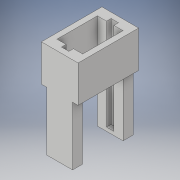
# Autodesk Inventor part: Colorimeter_Mounting-Tool
Saved by Autodesk Inventor 2019 (Build 230136000, 136)
## iProperties
Created: 2019-04-03
Part Number: Colorimeter_Mounting-Tool
Material: Generic
Document SubType Name: Modeling
Designer: Hansen
Density: 1 g/cm^3
Appearance: Default
Author: Hansen
Autodesk Inventor part; units mm, degrees
ref_plane "YZ Plane" through (0, 0, 0) normal (1, 0, 0) x (0, 1, 0)
ref_plane "XZ Plane" through (0, 0, 0) normal (0, 1, 0) x (-1, 0, 0)
ref_plane "XY Plane" through (0, 0, 0) normal (0, 0, 1) x (1, 0, 0)
sketch "Sketch1" plane through (0, 0, 0) normal (0, 1, 0) x (-1, 0, 0)
  line L0 (1, 6.75) -> (3.5, 6.75)
  line L1 (3.5, 6.75) -> (3.5, 5.5)
  line L2 (3.5, 5.5) -> (1, 5.5)
  line L3 (1, 5.5) -> (1, 6.75)
  line L4 (1, 6.75) -> (3.5, 5.5) construction
  line L5 (3.5, 6.75) -> (1, 5.5) construction
  line L6 (1, -5.5) -> (3.5, -5.5)
  line L7 (3.5, -5.5) -> (3.5, -6.75)
  line L8 (3.5, -6.75) -> (1, -6.75)
  line L9 (1, -6.75) -> (1, -5.5)
  line L10 (1, -5.5) -> (3.5, -6.75) construction
  line L11 (3.5, -5.5) -> (1, -6.75) construction
  line L12 (-1, 6.75) -> (-3.5, 6.75)
  line L13 (-3.5, 6.75) -> (-3.5, 5.5)
  line L14 (-3.5, 5.5) -> (-1, 5.5)
  line L15 (-1, 5.5) -> (-1, 6.75)
  line L16 (-1, 6.75) -> (-3.5, 5.5) construction
  line L17 (-3.5, 6.75) -> (-1, 5.5) construction
  line L18 (-1, -5.5) -> (-3.5, -5.5)
  line L19 (-3.5, -5.5) -> (-3.5, -6.75)
  line L20 (-3.5, -6.75) -> (-1, -6.75)
  line L21 (-1, -6.75) -> (-1, -5.5)
  line L22 (-1, -5.5) -> (-3.5, -6.75) construction
  line L23 (-3.5, -5.5) -> (-1, -6.75) construction
  line L24 (3.5, -6.75) -> (-3.5, -6.75)
  line L25 (-3.5, -6.75) -> (-3.5, -8.25)
  line L26 (-3.5, -8.25) -> (3.5, -8.25)
  line L27 (3.5, -8.25) -> (3.5, -6.75)
  line L28 (3.5, 6.75) -> (-3.5, 6.75)
  line L29 (-3.5, 6.75) -> (-3.5, 8.25)
  line L30 (-3.5, 8.25) -> (3.5, 8.25)
  line L31 (3.5, 8.25) -> (3.5, 6.75)
  point P0 (0, 0)
  point P1 (2.25, 6.125)
  point P2 (2.25, -6.125)
  point P3 (-2.25, 6.125)
  point P4 (-2.25, -6.125)
  point P5 (2.25, 6.125)
  point P6 (2.25, -6.125)
  point P7 (-2.25, 6.125)
  point P8 (-2.25, -6.125)
  point P9 (2.25, -6.125)
  point P10 (-2.25, -6.125)
  point P11 (2.25, 6.125)
  point P12 (-2.25, 6.125)
  dimension "d0" = 2
  dimension "d1" = 11
  dimension "d2" = 5.5
  dimension "d3" = 1
  dimension "d5" = 2.5
  dimension "d6" = 13.5
  dimension "d7" = 1.5
  constraints: 64 end point, 16 midpoint, 12 parallel, 6 horizontal, 6 perpendicular, 5 point on line, 3 collinear, 2 horizontal alignment, 2 vertical alignment, 1 coincident
  measures "d0" distance between parallel lines of L15 L3
  measures "d1" distance between parallel lines of L6 L2
  measures "d2" distance from line of point (0, 0) L2
  measures "d3" distance from line of point (0, 0) L15
  measures "d5" distance of L7.end L8.end
  measures "d6" distance between parallel lines of L8 L0
  measures "d7" distance of L26.end L7.end
extrude "Extrusion1" add sketch "Sketch1" against normal blind 25
sketch "Sketch2" plane through (0, 0, 0) normal (0, 1, 0) x (1, 0, 0)
  line L0 (3.5, 5.5) -> (3.5, 8.25) projected
  line L1 (3.5, 8.25) -> (5, 8.25)
  line L2 (5, 8.25) -> (5, -8.25)
  line L3 (5, -8.25) -> (3.5, -8.25)
  line L4 (3.5, -8.25) -> (3.5, 8.25)
  line L5 (-3.5, 8.25) -> (-3.5, 5.5) projected
  line L6 (-3.5, 8.25) -> (-5, 8.25)
  line L7 (-5, 8.25) -> (-5, -8.25)
  line L8 (-5, -8.25) -> (-3.5, -8.25)
  line L9 (-3.5, -8.25) -> (-3.5, 8.25)
  point P0 (0, 0)
  dimension "d10" = 1.5
  constraints: 16 end point, 4 parallel, 2 horizontal, 2 perpendicular, 1 coincident, 1 collinear, 1 point on line
  measures "d10" distance of L5.start L6.end
extrude "Extrusion2" add sketch "Sketch2" against normal blind 10
sketch "Sketch3" plane through (0, -25, 0) normal (0, -1, 0) x (1, 0, 0)
  line L0 (-3.5, 5.5) -> (-1, 5.5) projected
  line L1 (3.5, 5.5) -> (3.5, 8.25) projected
  line L2 (-3.5, 5.5) -> (3.5, 5.5)
  line L3 (3.5, 5.5) -> (3.5, 8.25)
  line L4 (3.5, 8.25) -> (-3.5, 8.25)
  line L5 (-3.5, 8.25) -> (-3.5, 5.5)
  line L6 (3.5, -5.5) -> (1, -5.5) projected
  line L7 (-3.5, -5.5) -> (-3.5, -8.25) projected
  line L8 (3.5, -5.5) -> (-3.5, -5.5)
  line L9 (-3.5, -5.5) -> (-3.5, -8.25)
  line L10 (-3.5, -8.25) -> (3.5, -8.25)
  line L11 (3.5, -8.25) -> (3.5, -5.5)
  point P0 (0, 0)
  constraints: 16 end point, 4 parallel, 2 horizontal, 2 perpendicular
extrude "Extrusion3" add sketch "Sketch3" along normal blind 1
equation "\"d2\" = 0.5 * d1"
equation "\"d3\" = 0.5 * d0"
body "Solid1"
